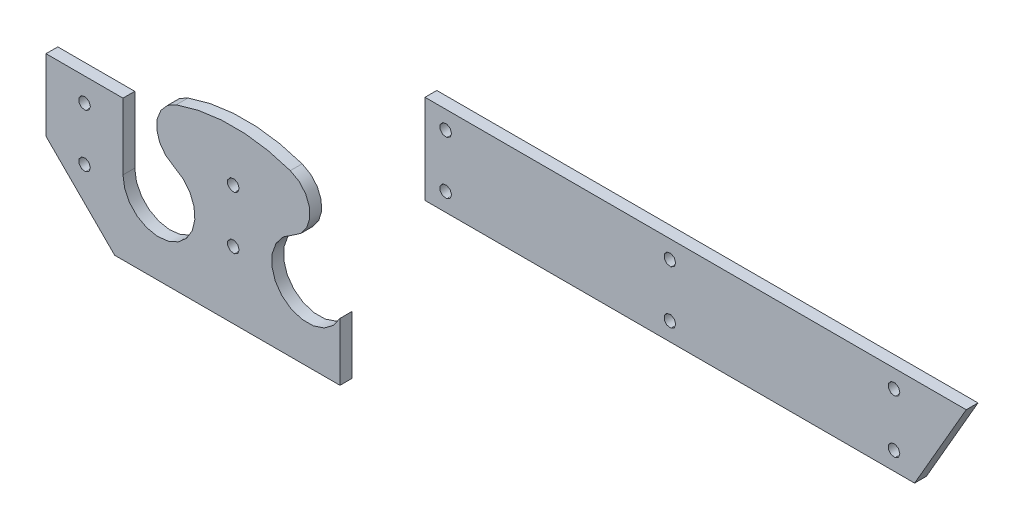
# Autodesk Inventor part: cierre carcasa
Saved by Autodesk Inventor 2017 (Build 210142000, 142)
## iProperties
Part Number: cierre carcasa
Material: Genérico
Document SubType Name: Modeling
Designer: Leo
Density: 1 g/cm^3
Appearance: Valor por defecto
Author: Leo
Autodesk Inventor part; units mm, degrees
ref_plane "YZ Plane" through (0, 0, 0) normal (1, 0, 0) x (0, 1, 0)
ref_plane "XZ Plane" through (0, 0, 0) normal (0, 1, 0) x (-1, 0, 0)
ref_plane "XY Plane" through (0, 0, 0) normal (0, 0, 1) x (1, 0, 0)
sketch "Boceto1" plane through (0, 0, 0) normal (0, 0, 1) x (1, 0, 0)
  circle A0 centre (224, 42.85) radius 2 projected
  circle A1 centre (72, 42.85) radius 2 projected
  circle A2 centre (0, -9.3174) radius 2 projected
  circle A3 centre (-50.45, -10.45) radius 2 projected
  circle A4 centre (224, 24.85) radius 2 projected
  circle A5 centre (72, 24.85) radius 2 projected
  circle A6 centre (0, -27.3174) radius 2 projected
  circle A7 centre (-50.45, -28.45) radius 2 projected
  arc A8 (18.9077, -14.5479) -> (36.1757, -30.3268) centre (25.2, -25) ccw projected
  arc A9 (-37.4, -25) -> (-18.9077, -14.5479) centre (-25.2, -25) ccw projected
  arc A10 (20.1441, -13.8969) -> (26, -4.796) centre (16, -4.796) ccw projected
  arc A11 (-26, -4.796) -> (-20.1441, -13.8969) centre (-16, -4.796) ccw projected
  arc A12 (20.1441, -13.8969) -> (18.9077, -14.5479) centre (25.2, -25) ccw
  arc A13 (-18.9077, -14.5479) -> (-20.1441, -13.8969) centre (-25.2, -25) ccw
  arc A14 (-19.3367, 4.6309) -> (-26, -4.796) centre (-16, -4.796) ccw
  arc A15 (19.3367, 4.6309) -> (-19.3367, 4.6309) centre (0, -50) ccw
  arc A16 (26, -4.796) -> (19.3367, 4.6309) centre (16, -4.796) ccw
  line L0 (-37.4, -25) -> (-37.4, -2.45)
  line L1 (-37.4, -2.45) -> (-63.5, -2.45)
  line L2 (-63.5, -2.45) -> (-63.5, -26.7137)
  line L3 (-40.2137, -50) -> (36.1757, -50)
  line L4 (36.1757, -50) -> (36.1757, -30.3268)
  line L5 (-63.5, -26.7137) -> (-40.2137, -50)
  line L6 (276.8, -56) -> (-78.2, -56) projected
  circle A17 centre (148, 42.85) radius 2 projected
  circle A18 centre (148, 24.85) radius 2 projected
  line L7 (248.4937, 49) -> (65, 49)
  line L8 (65, 49) -> (65, 18.7)
  line L9 (65, 18.7) -> (231, 18.7)
  line L10 (231, 18.7) -> (248.4937, 49)
  line L11 (-78.2, 56) -> (276.8, 56) projected
  line L12 (72, 24.85) -> (72, 42.85) construction
  point P0 (0, 0)
  point P1 (-50.45, -2.45)
  point P2 (72, 33.85)
  point P3 (65, 33.85)
  point P4 (148, 18.7)
  dimension "d0" = 13.05
  dimension "d1" = 45
  dimension "d2" = 6
  dimension "d3" = 8
  dimension "d4" = 6
  dimension "d5" = 7
  dimension "d6" = 120
  dimension "d7" = 5
  constraints: 22 end point, 10 point on circle, 8 tangent, 7 perpendicular, 5 centre point, 4 midpoint, 2 equal radius, 2 vertical alignment, 1 horizontal, 1 horizontal alignment, 1 point on line, 1 vertical
  measures "d0" distance from line of L2 A3.centre
  measures "d1" angle of L5 L3
  measures "d2" distance edge to line of A7 L5
  measures "d3" distance from line of A3.centre L1
  measures "d4" distance between parallel lines of L3 L6
  measures "d5" distance between parallel lines of L11 L7
  measures "d6" angle of L10 L9
  measures "d7" distance edge to line of A1 L8
extrude "Extrusión1" add sketch "Boceto1" along normal blind 4
